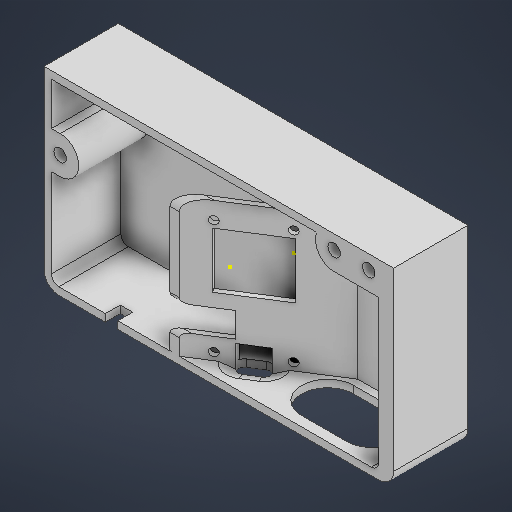
# Autodesk Inventor part: 后盖电路
Saved by Autodesk Inventor 2025 (Build 290162000, 162)
## iProperties
Created: 2025-12-26
Part Number: 后盖电路
Material: 常规
Document SubType Name: Modeling
Designer: XH
Density: 1 g/cm^3
Appearance: 默认
Author: XH
Autodesk Inventor part; units mm, degrees
ref_plane "YZ Plane" through (0, 0, 0) normal (1, 0, 0) x (0, 1, 0)
ref_plane "XZ Plane" through (0, 0, 0) normal (0, 1, 0) x (-1, 0, 0)
ref_plane "XY Plane" through (0, 0, 0) normal (0, 0, 1) x (1, 0, 0)
sketch "草图1" plane through (0, 0, 0) normal (0, 0, 1) x (1, 0, 0)
  line L0 (-69.1834, -44.3704) -> (56.8166, -44.3704)
  arc A0 (56.8166, -44.3704) -> (62.8166, -38.3704) centre (56.8166, -38.3704) ccw
  line L1 (62.8166, 27.5796) -> (62.8166, -38.3704)
  line L2 (62.8166, 27.5796) -> (62.8166, 32.6296)
  line L3 (62.8166, 32.6296) -> (-75.1834, 32.6296)
  line L4 (-75.1834, -38.3704) -> (-75.1834, 32.6296)
  arc A1 (-75.1834, -38.3704) -> (-69.1834, -44.3704) centre (-69.1834, -38.3704) ccw
  constraints: 10 end point, 4 point on circle, 2 centre point, 2 other
extrude "拉伸1" add sketch "草图1" along normal blind 30
sketch "草图2" plane through (0, 0, 30) normal (0, 0, 1) x (1, 0, 0)
  point P0 (0, 0)
sketch "草图3" plane through (0, 0, 30) normal (0, 0, 1) x (1, 0, 0)
  line L0 (-69.1834, -44.3704) -> (56.8166, -44.3704) projected
  arc A0 (-75.1834, -38.3704) -> (-69.1834, -44.3704) centre (-69.1834, -38.3704) ccw projected
  line L1 (-75.1834, 32.6296) -> (-75.1834, -38.3704) projected
  line L2 (62.8166, 32.6296) -> (-75.1834, 32.6296) projected
  line L3 (62.8166, -38.3704) -> (62.8166, 32.6296) projected
  arc A1 (56.8166, -44.3704) -> (62.8166, -38.3704) centre (56.8166, -38.3704) ccw projected
  line L4 (-69.1834, -41.3704) -> (56.8166, -41.3704)
  arc A2 (56.8166, -41.3704) -> (59.8166, -38.3704) centre (56.8166, -38.3704) ccw
  line L5 (59.8166, -38.3704) -> (59.8166, 29.6296)
  line L6 (59.8166, 29.6296) -> (-72.1834, 29.6296)
  line L7 (-72.1834, 29.6296) -> (-72.1834, -38.3704)
  arc A3 (-72.1834, -38.3704) -> (-69.1834, -41.3704) centre (-69.1834, -38.3704) ccw
  point P0 (0, 0)
  dimension "d3" = 3
  constraints: 8 end point, 4 point on circle, 2 centre point, 5 other
  measures "d3" radial gap between concentric circles of A0 A3
extrude "拉伸2" cut sketch "草图3" against normal blind 28 contours A3 L7 L6 L5 A2 L4
move faces "移动1" translate (3, 0, 0) faces at (62.8166, 29.263, 10) (62.8166, -16.387, 10) (59.0087, -43.9556, 20)
sketch "草图4" plane through (-69.1834, -44.3704, 0) normal (0, -1, 0) x (1, 0, 0)
  line L0 (23.7545, 33.1921) -> (18.7545, 33.1921) projected
  line L1 (23.7545, 33.1921) -> (18.7545, 33.1921)
  line L2 (18.7545, 33.1921) -> (18.7545, 24)
  line L3 (18.7545, 24) -> (23.7545, 24)
  line L4 (23.7545, 24) -> (23.7545, 33.1921)
  line L5 (0, 30) -> (129, 30) projected
  point P0 (69.1834, 0)
  point P1 (21.2545, 24)
  point P2 (18.7545, 33.1921)
  dimension "d9" = 6
  constraints: 8 end point, 2 parallel, 1 horizontal, 1 midpoint, 1 perpendicular
  measures "d9" distance from line of L5 point (21.254, 24)
extrude "拉伸3" cut sketch "草图4" against normal blind 10
sketch "草图5" plane through (0, 0, 0) normal (0, 0, -1) x (-1, 0, 0)
  circle A0 centre (-55.8166, 26.9427) radius 2.5 projected
  circle A1 centre (-41.8166, 26.9427) radius 2.5 projected
  circle A2 centre (68.6834, 4.8796) radius 2.5 projected
  circle A3 centre (68.6834, 4.8796) radius 4.5
  circle A4 centre (-41.8166, 26.9427) radius 4.5
  circle A5 centre (-55.8166, 26.9427) radius 4.5
  point P0 (0, 0)
  dimension "d12" = 2
  dimension "d13" = 2
  dimension "d14" = 2
  constraints: 3 centre point
  measures "d12" radial gap between concentric circles of A2 A3
  measures "d13" radial gap between concentric circles of A1 A4
  measures "d14" radial gap between concentric circles of A0 A5
extrude "拉伸4" cut sketch "草图5" against normal blind 110.5 contours A0 | A1 | A2 | A3 | A4 | A5
sketch "草图6" plane through (0, 0, 2) normal (0, 0, 1) x (1, 0, 0)
  arc A0 (38.2068, 29.6296) -> (45.4264, 29.6296) centre (41.8166, 26.9427) ccw projected
  circle A1 centre (41.8166, 26.9427) radius 4.5
  circle A2 centre (41.8166, 26.9427) radius 2.5 projected
  circle A3 centre (55.8166, 26.9427) radius 2.5 projected
  circle A4 centre (55.8166, 26.9427) radius 4.5
  circle A5 centre (-68.6834, 4.8796) radius 4.5 projected
  circle A6 centre (-68.6834, 4.8796) radius 4.5
  circle A7 centre (-68.6834, 4.8796) radius 2.5 projected
  point P0 (0, 0)
  point P1 (45.4264, 29.6296)
  constraints: 3 centre point, 3 coincident
extrude "拉伸5" add sketch "草图6" along normal up to surface (28 mm away)
delete faces "删除1" heal yes whole lump no faces at (59.6866, 29.6296, 20.6667)
sketch "草图7" plane through (0, 0, 2) normal (0, 0, 1) x (1, 0, 0)
  arc A0 (-72.1834, 2.0512) -> (-72.1834, 7.7081) centre (-68.6834, 4.8796) ccw projected
  line L0 (-68.6834, 9.3796) -> (-72.1834, 9.3796)
  line L1 (-72.1834, 7.7081) -> (-72.1834, 29.6296) projected
  line L2 (-68.6834, 4.8796) -> (-61.8258, 4.8796)
  line L3 (-68.6834, 0.3796) -> (-72.1834, 0.3796)
  line L4 (-72.1834, -38.3704) -> (-72.1834, 2.0512) projected
  point P0 (0, 0)
  constraints: 6 end point, 2 symmetric about line, 1 horizontal, 1 perpendicular, 1 point on circle, 1 point on line
extrude "拉伸6" add sketch "草图7" along normal up to surface (28 mm away)
sketch "草图8" plane through (0, 0, 2) normal (0, 0, 1) x (1, 0, 0)
  arc A0 (38.2068, 29.6296) -> (45.4264, 29.6296) centre (41.8166, 26.9427) ccw projected
  line L0 (41.8166, 22.4427) -> (55.8166, 22.4427)
  arc A1 (52.2068, 29.6296) -> (59.8166, 24.8812) centre (55.8166, 26.9427) ccw projected
  line L1 (-72.1834, 9.3796) -> (-68.6834, 9.3796) projected
  arc A2 (-68.6834, 0.3796) -> (-68.6834, 9.3796) centre (-68.6834, 4.8796) ccw projected
  line L2 (-68.6834, 0.3796) -> (-72.1834, 0.3796) projected
  line L3 (-72.1834, -38.3704) -> (-72.1834, 0.3796) projected
  arc A3 (-72.1834, -38.3704) -> (-69.1834, -41.3704) centre (-69.1834, -38.3704) ccw projected
  line L4 (56.8166, -41.3704) -> (-69.1834, -41.3704) projected
  arc A4 (56.8166, -41.3704) -> (59.8166, -38.3704) centre (56.8166, -38.3704) ccw projected
  line L5 (59.8166, 24.8812) -> (59.8166, -38.3704) projected
  arc A5 (52.2068, 29.6296) -> (59.8166, 24.8812) centre (55.8166, 26.9427) ccw projected
  line L6 (45.4264, 29.6296) -> (52.2068, 29.6296) projected
  arc A6 (38.2068, 29.6296) -> (45.4264, 29.6296) centre (41.8166, 26.9427) ccw projected
  line L7 (-72.1834, 29.6296) -> (38.2068, 29.6296) projected
  line L8 (-72.1834, 9.3796) -> (-72.1834, 29.6296) projected
  point P0 (0, 0)
  point P1 (45.4264, 29.6296)
  constraints: 2 end point, 2 point on circle, 1 horizontal
extrude "拉伸7" add sketch "草图8" along normal up to surface (28 mm away) contours A0 L6 A1 L0
delete faces "删除2" heal yes whole lump no faces at (41.8166, 22.4427, 0.6667) (52.5269, 30.0132, 1.3333) (39.0332, 29.5465, 2) (59.4203, 25.7174, 2) (-66.5182, 1.7429, 2) (-68.141, 9.3468, 1.3333)
delete faces "删除3" heal yes whole lump no faces at (57.1119, 22.6332, 20.6667)
offset faces "大小1" outward 3 faces at (-69.85, 9.3796, 11.3333) (-68.3213, 9.365, 20.6667) (-71.0167, 0.3796, 11.3333)
offset faces "大小2" outward 3 faces at (47.8166, 22.4427, 20.6667) (41.4486, 22.4578, 20.6667)
sketch "草图9" plane through (-72.1834, 29.6296, 2) normal (0, -1, 0) x (1, 0, 0)
  line L0 (138, 28) -> (-3, 28) projected
  line L1 (47.8065, 28) -> (94.9823, -2)
  line L2 (138, -2) -> (-3, -2) projected
  line L3 (55.6477, 17.7868) -> (31.1766, 33.3484)
  line L4 (51.5336, 28) -> (98.7094, -2)
  point P0 (72.1834, -2)
  dimension "d25" = 2
  constraints: 6 end point, 4 point on line, 2 parallel, 3 other
  measures "d25" distance between parallel lines of L1 L4
extrude "拉伸8" add sketch "草图9" along normal up to surface (74 mm away)
sketch "草图10" plane through (23.381, -41.3704, 2) normal (0.5366089, 0, 0.8438311) x (0.8438311, 0, -0.5366089)
  point P0 (-18.6564, 41.3704)
sketch "草图11" plane through (23.381, -41.3704, 2) normal (0.5366089, 0, 0.8438311) x (0.8438311, 0, -0.5366089)
  line L0 (0, 0) -> (-52.1795, 0) projected
  line L1 (0, 71) -> (0, 0) projected
  line L2 (-52.1795, 71) -> (0, 71) projected
  line L3 (-52.1795, 71) -> (-52.1795, 0) projected
  line L4 (-55.3246, 0) -> (-3.1451, 0) projected
  line L5 (-42.724, 71) -> (0, 71)
  line L6 (-52.1795, 71) -> (0, 71) projected
  line L7 (0, 71) -> (-40, 71)
  line L8 (-40, 71) -> (-40, 56)
  line L9 (-40, 56) -> (0, 56)
  line L10 (0, 56) -> (0, 71)
  point P0 (-18.6564, 41.3704)
  point P1 (0, 56)
  point P2 (-40, 71)
  dimension "d36" = 40
  dimension "d37" = 15
  constraints: 10 end point, 2 parallel, 2 perpendicular, 1 collinear, 1 horizontal, 1 point on line
  measures "d36" distance of L8.end L9.end
  measures "d37" distance of L7.end L8.end
extrude "拉伸9" cut sketch "草图11" against normal up to surface (2 mm away) contours L9 L8 L2 L1
sketch "草图12" plane through (-50.4289, -44.3704, 24) normal (0, -1, 0) x (1, 0, 0)
  arc A0 (93.1716, -18) -> (93.1716, 1) centre (93.1716, -8.5) ccw
  line L0 (75.1716, 1) -> (93.1716, 1)
  arc A1 (75.1716, 1) -> (75.1716, -18) centre (75.1716, -8.5) ccw
  line L1 (93.1716, -18) -> (75.1716, -18)
  arc A2 (75.1716, 2) -> (75.1716, -19) centre (75.1716, -8.5) ccw
  line L2 (75.1716, 2) -> (93.1716, 2)
  arc A3 (93.1716, -19) -> (93.1716, 2) centre (93.1716, -8.5) ccw
  line L3 (93.1716, -19) -> (75.1716, -19)
  line L4 (-18.7545, -24) -> (110.2455, -24) projected
  point P0 (50.4289, -24)
  dimension "d38" = 1
  dimension "d39" = 9.5
  dimension "d40" = 19
  dimension "d41" = 9.5
  dimension "d42" = 6
  constraints: 8 end point, 8 point on circle, 4 centre point, 3 other
  measures "d38" radial gap between concentric circles of A1 A2
  measures "d39" radius of A1
  measures "d40" distance between parallel lines of L1 L0
  measures "d41" radius of A0
  measures "d42" distance between parallel lines of L4 L1
extrude "拉伸10" cut sketch "草图12" against normal up to surface (63.8131 mm away) contours L1 A1 L0 A0 | L2 A3 L3 A2
delete faces "删除5" heal yes whole lump no faces at (20.5385, 24.6296, 1.4374) (22.6655, 24.6296, 0.8749)
sketch "草图13" plane through (-20.6497, -41.3704, 30) normal (0.5366089, 0, 0.8438311) x (0.8438311, 0, -0.5366089)
  circle A0 centre (10.1121, 49.0796) radius 1.5875 projected
  circle A1 centre (33.4371, 49.0796) radius 1.5875 projected
  circle A2 centre (33.4371, 3.0421) radius 1.5875 projected
  circle A3 centre (10.1121, 3.0421) radius 1.5875 construction
  circle A4 centre (10.1121, 3.0421) radius 1.5875 projected
  line L0 (9.7246, 51.9546) -> (34.0246, 51.9546) projected
  line L1 (7.7246, 2.4546) -> (7.7246, 49.9546) projected
  arc A5 (9.7246, 51.9546) -> (7.7246, 49.9546) centre (9.7246, 49.9546) ccw projected
  arc A6 (36.0246, 49.9546) -> (34.0246, 51.9546) centre (34.0246, 49.9546) ccw projected
  line L2 (36.0246, 49.9546) -> (36.0246, 2.4546) projected
  line L3 (21.8746, 51.9546) -> (21.8746, 15.0021)
  line L4 (34.0246, 23.8346) -> (9.7246, 23.8346)
  line L5 (9.7246, 23.8346) -> (9.7246, 46.274)
  line L6 (9.7246, 46.274) -> (34.0246, 46.274)
  line L7 (34.0246, 46.274) -> (34.0246, 23.8346)
  line L8 (34.0246, 23.8346) -> (9.7246, 46.274) construction
  line L9 (9.7246, 23.8346) -> (34.0246, 46.274) construction
  point P0 (33.5231, 41.3704)
  point P1 (21.8746, 35.0543)
  constraints: 14 end point, 3 midpoint, 2 parallel, 1 horizontal, 1 perpendicular, 1 point on line, 1 vertical
extrude "拉伸11" cut sketch "草图13" against normal blind 10
sketch "草图14" plane through (-50.4289, -44.3704, 24) normal (0, -1, 0) x (1, 0, 0)
  line L0 (51.3178, -6.2521) -> (46.4658, -3.1666)
  arc A0 (46.4658, -3.1666) -> (44.7218, -5.9091) centre (45.5938, -4.5378) ccw
  arc A1 (49.5739, -8.9946) -> (51.3178, -6.2521) centre (50.4458, -7.6233) ccw
  line L1 (44.8291, -5.7403) -> (49.6812, -8.8258)
  line L2 (75.1716, 2) -> (93.1716, 2) construction
  arc A2 (93.1716, -19) -> (93.1716, 2) centre (93.1716, -8.5) ccw construction
  line L3 (93.1716, -19) -> (75.1716, -19) construction
  arc A3 (75.1716, 2) -> (75.1716, -19) centre (75.1716, -8.5) ccw construction
  line L4 (5, 6) -> (110.2455, 6) construction
  line L5 (5, 6) -> (5, 0) construction
  line L6 (5, 0) -> (0, 0) construction
  line L7 (0, 0) -> (0, 6) construction
  line L8 (-18.7545, 6) -> (0, 6) construction
  line L9 (-18.7545, -24) -> (-18.7545, 6) construction
  line L10 (-18.7545, -24) -> (110.2455, -24) construction
  line L11 (110.2455, 6) -> (110.2455, -24) construction
  line L12 (44.7218, -5.9091) -> (49.5739, -8.9946) construction
  line L13 (44.8291, -5.7403) -> (49.6812, -8.8258) construction
  line L14 (44.7218, -5.9091) -> (49.5739, -8.9946)
  line L15 (46.9333, -2.4315) -> (51.7853, -5.517)
  arc A4 (49.1064, -9.7296) -> (51.7853, -5.517) centre (50.4458, -7.6233) ccw
  line L16 (49.1064, -9.7296) -> (44.2544, -6.6441)
  arc A5 (46.9333, -2.4315) -> (44.2544, -6.6441) centre (45.5938, -4.5378) ccw
  point P0 (50.4289, -24)
extrude "拉伸12" cut sketch "草图14" against normal blind 10 contours A1 L14 A0 L0 | L15 A4 L16 A5
sketch "草图15" plane through (-20.6497, -41.3704, 30) normal (0.5366089, 0, 0.8438311) x (0.8438311, 0, -0.5366089)
  line L0 (6.5414, 18.5081) -> (-5.3759, 18.5081)
  line L1 (-5.3759, 18.5081) -> (-5.3759, 8.5081)
  line L2 (-5.3759, 8.5081) -> (6.5414, 8.5081)
  line L3 (6.5414, 8.5081) -> (6.5414, 18.5081)
  line L4 (6.5414, 18.5081) -> (-5.3759, 8.5081) construction
  line L5 (-5.3759, 18.5081) -> (6.5414, 8.5081) construction
  point P0 (33.5231, 41.3704)
  point P1 (0.5827, 13.5081)
  dimension "d49" = 10
  constraints: 12 end point, 2 midpoint, 2 parallel, 1 horizontal, 1 perpendicular
  measures "d49" distance of L0.end L1.end
extrude "拉伸13" cut sketch "草图15" against normal blind 10
fillet "圆角1" radius 2 2 edges at (-22.5133, -32.8622, 30) (-22.5133, -22.8622, 30)
chamfer "倒角1" distance 5 distance2 2 3 edges at (-1.0697, -41.3704, 20.0257) (-5.1768, -41.3704, 21.9348) (2.4011, -41.3704, 17.1159) measured on face at (2.8786, -41.3704, 17.2639) measured on face at (-0.8013, -41.3704, 20.4476) measured on face at (-5.2452, -41.3704, 22.4301)
delete faces "删除6" heal yes whole lump no faces at (-11.0877, 24.6296, 22.3392)
fillet "圆角2" radius 5.5 1 edges at (-22.5133, 14.6296, 30)
move faces "移动5" translate (8.4383, 0, -5.3661) faces at (-15.4876, -29.5289, 25.9273)
